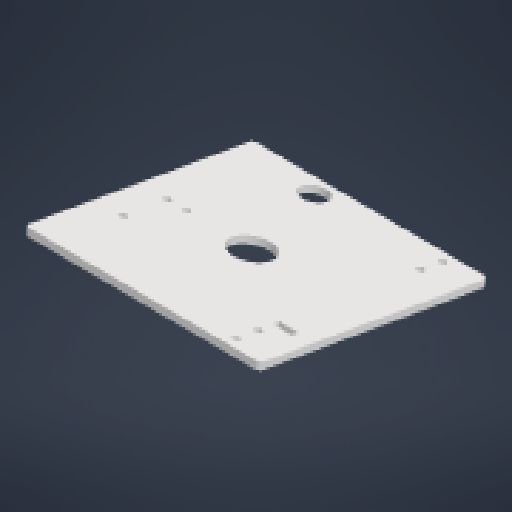
# Autodesk Inventor part: BaseMotoJose
Saved by Autodesk Inventor 2026.3 (Build 303398000, 398)
## iProperties
Created: 2026-04-28
Part Number: BaseMotoJose
Material: Genérico
Document SubType Name: Modeling
Designer: Jose Carlos
Density: 1 g/cm^3
Appearance: Valor por defecto
Author: Jose Carlos
Autodesk Inventor part; units mm, degrees
ref_plane "YZ Plane" through (0, 0, 0) normal (1, 0, 0) x (0, 1, 0)
ref_plane "XZ Plane" through (0, 0, 0) normal (0, 1, 0) x (-1, 0, 0)
ref_plane "Plano de trabajo1" through (39.4603, 28.9326, 43.4345) normal (-0.0230448, -0.9802565, 0.1963824) x (0.9993754, -0.0278517, -0.0217506)
sketch "Boceto1" plane through (39.4603, 28.9326, 43.4345) normal (-0.0230448, -0.9802565, 0.1963824) x (0.9993754, -0.0278517, -0.0217506)
  circle A0 centre (25.7474, -0.0015) radius 6 construction
  circle A1 centre (25.7474, -0.0015) radius 8.5 construction
  circle A2 centre (25.7474, -0.0015) radius 8.5
  line L0 (73.7302, -52.0094) -> (-22.2354, -52.0094)
  line L1 (-22.2354, -52.0094) -> (-22.2354, 52.0063)
  line L2 (-22.2354, 52.0063) -> (73.7302, 52.0063)
  line L3 (73.7302, 52.0063) -> (73.7302, -52.0094)
  line L4 (73.7302, -52.0094) -> (-22.2354, 52.0063) construction
  line L5 (-22.2354, -52.0094) -> (73.7302, 52.0063) construction
  line L6 (18.0272, 52.0081) -> (-18.0728, 52.0046) construction
  line L7 (73.7311, 10.0133) -> (73.7292, 30.0133) construction
  circle A3 centre (11.587, -43.5711) radius 5.65 construction
  circle A4 centre (11.587, -43.5711) radius 5.65
  line L8 (77.9675, -50.0094) -> (77.9675, 50.0063) projected
  line L9 (73.7302, 52.0063) -> (77.9675, 52.0063)
  line L10 (77.9675, 52.0063) -> (77.9675, -52.0094)
  line L11 (77.9675, -52.0094) -> (73.7302, -52.0094)
  line L12 (73.7302, -52.0094) -> (73.7302, 52.0063)
  line L13 (77.9675, 17.0063) -> (74.9675, 17.0063) projected
  line L14 (77.9675, 37.0063) -> (74.9675, 37.0063) projected
  line L15 (77.9675, -37.0094) -> (74.9675, -37.0094) projected
  line L16 (77.9675, -17.0094) -> (74.9675, -17.0094) projected
  line L17 (77.9675, -37.0094) -> (73.7302, -37.0094)
  line L18 (73.7302, -37.0094) -> (73.7302, -17.0094)
  line L19 (73.7302, -17.0094) -> (77.9675, -17.0094)
  line L20 (77.9675, -17.0094) -> (77.9675, -37.0094)
  line L21 (77.9675, 17.0063) -> (73.7302, 17.0063)
  line L22 (73.7302, 17.0063) -> (73.7302, 37.0063)
  line L23 (73.7302, 37.0063) -> (77.9675, 37.0063)
  line L24 (77.9675, 37.0063) -> (77.9675, 17.0063)
  line L25 (77.9675, 52.0063) -> (80.9675, 52.0063)
  line L26 (80.9675, 52.0063) -> (80.9675, 37.0063)
  line L27 (80.9675, 37.0063) -> (77.9675, 37.0063)
  line L28 (77.9675, 37.0063) -> (77.9675, 52.0063)
  line L29 (77.9675, 17.0063) -> (80.9675, 17.0063)
  line L30 (80.9675, 17.0063) -> (80.9675, -17.0094)
  line L31 (80.9675, -17.0094) -> (77.9675, -17.0094)
  line L32 (77.9675, -17.0094) -> (77.9675, 17.0063)
  line L33 (77.9675, -37.0094) -> (80.9675, -37.0094)
  line L34 (80.9675, -37.0094) -> (80.9675, -52.0094)
  line L35 (80.9675, -52.0094) -> (77.9675, -52.0094)
  line L36 (77.9675, -52.0094) -> (77.9675, -37.0094)
  point P0 (-37.6851, -49.2992)
  point P1 (73.7302, 20.0133)
  point P2 (-0.0228, 52.0063)
  point P3 (77.9675, -0.0015)
  point P4 (76.4675, -17.0094)
  point P5 (77.9675, -50.0094)
  point P6 (74.9675, -37.0094)
  point P7 (74.9675, 17.0063)
  point P8 (73.7302, 17.0063)
  point P9 (73.7302, -17.0094)
  point P10 (74.9675, -17.0094)
  point P11 (73.7302, 37.0063)
  point P12 (74.9675, 37.0063)
  point P13 (77.9675, 50.0063)
  point P14 (77.9675, -52.0094)
  point P15 (77.9675, -17.0094)
  point P16 (77.9675, 37.0063)
  dimension "d33" = 3
  constraints: 60 end point, 14 parallel, 8 point on line, 7 horizontal, 7 midpoint, 7 perpendicular, 2 centre point, 2 coincident, 2 concentric
  measures "d33" distance of L9.end L25.end
extrude "Extrusión1" add sketch "Boceto1" along normal blind 3
sketch "Boceto3" plane through (39.3912, 25.9918, 44.0236) normal (-0.0230448, -0.9802565, 0.1963824) x (0.9993754, -0.0278517, -0.0217506)
  line L0 (44.9302, -50.0094) -> (44.9302, 50.0063) construction
  line L1 (47.9302, -50.0094) -> (47.9302, 50.0063) construction
  line L2 (44.9302, 37.0063) -> (47.9302, 37.0063)
  line L3 (47.9302, 37.0063) -> (47.9302, 17.0063)
  line L4 (47.9302, 17.0063) -> (44.9302, 17.0063)
  line L5 (44.9302, 17.0063) -> (44.9302, 37.0063)
  line L6 (73.7302, 52.0063) -> (-22.2354, 52.0063) construction
  line L7 (44.9302, -17.0094) -> (47.9302, -17.0094)
  line L8 (47.9302, -17.0094) -> (47.9302, -37.0094)
  line L9 (47.9302, -37.0094) -> (44.9302, -37.0094)
  line L10 (44.9302, -37.0094) -> (44.9302, -17.0094)
  line L11 (-22.2354, -52.0094) -> (73.7302, -52.0094) construction
  point P0 (-37.6851, -49.2992)
  point P1 (-22.2354, 52.0063)
  point P2 (-22.2354, -52.0094)
  point P3 (73.7302, -52.0094)
  point P4 (46.4302, -37.0094)
  dimension "d2" = 20
  dimension "d3" = 15
  dimension "d4" = 15
  dimension "d5" = 20
  constraints: 16 end point, 4 parallel, 4 point on line, 2 horizontal, 2 perpendicular, 1 midpoint, 2 other
  measures "d2" distance between parallel lines of L2 L4
  measures "d5" distance of L7.end L8.end
extrude "Extrusión2" [suppressed]
sketch "Boceto4" plane through (39.3912, 25.9918, 44.0236) normal (-0.0230448, -0.9802565, 0.1963824) x (0.9993754, -0.0278517, -0.0217506)
  circle A0 centre (62.9302, -47.0094) radius 1.6 construction
  circle A1 centre (62.9302, -37.0094) radius 1.6 construction
  circle A2 centre (62.9302, 37.0063) radius 1.6 construction
  circle A3 centre (62.9302, 47.0063) radius 1.6 construction
  point P0 (-37.6851, -49.2992)
hole "Agujero1" at (101.0227, 15.0366, -3.4278) at (101.2906, 16.9942, 6.3751) at (103.2735, 31.4834, 78.9317) at (103.5414, 33.441, 88.7345) direction (0.0230448, 0.9802565, -0.1963824) diameter 3 end through all
sketch "Boceto5" plane through (39.3912, 25.9918, 44.0236) normal (-0.0230448, -0.9802565, 0.1963824) x (0.9993754, -0.0278517, -0.0217506)
  line L0 (-22.2354, 52.0063) -> (-22.2354, -52.0094) construction
  line L1 (-22.2354, -52.0094) -> (73.7302, -52.0094) construction
  circle A0 centre (-10.3398, 19.9988) radius 1.6 construction
  circle A1 centre (-10.3398, -0.0012) radius 1.6 construction
  point P0 (-37.6851, -49.2992)
  point P1 (-2.2354, -0.0015)
  point P2 (-22.2354, -0.0015)
  dimension "d16" = 20
  dimension "d18" = 0
  constraints: 1 midpoint
  measures "d16" distance from line of L0 point (-2.235, -0.002)
  measures "d18" vertical distance of point (-22.235, -0.002) point (-2.235, -0.002)
hole "Agujero2" at (37.1571, 26.0538, 44.0708) at (29.5936, 30.1947, 63.853) at (29.0578, 26.2796, 44.2473) direction (0.0230448, 0.9802565, -0.1963824) diameter 3 end through all
sketch "Boceto6" plane through (39.3912, 25.9918, 44.0236) normal (-0.0230448, -0.9802565, 0.1963824) x (0.9993754, -0.0278517, -0.0217506)
  line L0 (70.7302, 30.0063) -> (62.7302, 30.0063)
  line L1 (62.7302, 30.0063) -> (62.7302, 27.0063)
  line L2 (62.7302, 27.0063) -> (70.7302, 27.0063)
  line L3 (70.7302, 27.0063) -> (70.7302, 30.0063)
  line L4 (70.7302, 30.0063) -> (62.7302, 27.0063) construction
  line L5 (62.7302, 30.0063) -> (70.7302, 27.0063) construction
  line L6 (73.7302, 17.0063) -> (73.7302, 37.0063) construction
  line L7 (73.7302, 52.0063) -> (-22.2354, 52.0063) construction
  point P0 (-37.6851, -49.2992)
  point P1 (66.7302, 28.5063)
  point P2 (73.7302, -52.0094)
  point P3 (70.7302, 28.5063)
  dimension "d26" = 8
  dimension "d27" = 3
  dimension "d28" = 3
  dimension "d29" = 22
  constraints: 12 end point, 3 midpoint, 2 parallel, 1 horizontal, 1 perpendicular
  measures "d26" distance of L0.start L0.end
  measures "d27" distance of L2.end L0.start
  measures "d28" distance from line of L6 point (70.73, 28.506)
  measures "d29" distance between parallel lines of L7 L0
extrude "Extrusión3" cut sketch "Boceto6" against normal through all
fillet "Empalme1" radius 2 8 edges at (18.5975, 38.2622, 95.1938) (15.8108, 17.9002, -6.7714) (121.736, 35.3878, 92.9491) (121.3341, 32.4514, 78.2448) (120.7983, 28.5363, 58.6391) (119.887, 21.8774, 25.2939) (119.3512, 17.9622, 5.6882) (118.9493, 15.0258, -9.0161)
